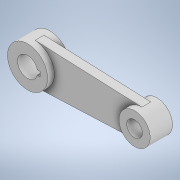
# Autodesk Inventor part: Biela da Valvula
Saved by Autodesk Inventor 2020 (Build 240168000, 168)
## iProperties
Created: 2022-04-28
Part Number: Biela da Valvula
Material: Genérico
Document SubType Name: Modeling
Designer: robofei
Density: 1 g/cm^3
Appearance: Padrão
Author: robofei
Autodesk Inventor part; units mm, degrees
ref_plane "YZ Plane" through (0, 0, 0) normal (1, 0, 0) x (0, 1, 0)
ref_plane "XZ Plane" through (0, 0, 0) normal (0, 1, 0) x (-1, 0, 0)
ref_plane "XY Plane" through (0, 0, 0) normal (0, 0, 1) x (1, 0, 0)
sketch "Esboço1" plane through (0, 0, 0) normal (0, 0, 1) x (1, 0, 0)
  circle A0 centre (0, 0) radius 21.9
  circle A1 centre (0, 0) radius 43.75
  arc A2 (-272.718, 6.3) -> (-272.718, -6.3) centre (-300, 0) ccw
  circle A3 centre (-300, 0) radius 56.25
  line L0 (-272.718, 6.3) -> (-265, 6.3)
  line L1 (-265, 6.3) -> (-265, -6.3)
  line L2 (-265, -6.3) -> (-272.718, -6.3)
  dimension "d0" = 300
  dimension "d1" = 87.5
  dimension "d2" = 43.8
  dimension "d3" = 112.5
  dimension "d4" = 56
  dimension "d6" = 12.6
  dimension "d7" = 6.3
  dimension "d8" = 35
  constraints: 6 end point, 4 centre point, 3 coincident, 2 point on circle, 1 horizontal, 1 parallel, 1 perpendicular
  measures "d0" distance of A2.centre point (0, 0)
  measures "d1" diameter of A1
  measures "d2" diameter of A0
  measures "d3" diameter of A3
  measures "d4" diameter of A2
  measures "d6" distance of L0.end L1.end
  measures "d7" distance from line of A2.centre L2
  measures "d8" horizontal distance of A2.centre L1.end
extrude "Extrusão1" add sketch "Esboço1" along normal mid plane 62.5
sketch "Esboço2" plane through (0, 0, 0) normal (0, 0, 1) x (1, 0, 0)
  arc A0 (1.8229, 43.712) -> (1.8229, -43.712) centre (0, 0) ccw
  arc A1 (-272.718, 6.3) -> (-272.718, -6.3) centre (-300, 0) ccw projected
  arc A2 (-297.6562, -56.2012) -> (-297.6562, 56.2012) centre (-300, 0) ccw
  line L0 (-297.6562, 56.2012) -> (1.8229, 43.712)
  line L1 (-297.6562, -56.2012) -> (1.8229, -43.712)
  circle A3 centre (0, 0) radius 43.75 projected
  circle A4 centre (-300, 0) radius 56.25 projected
  dimension "d11" = 87.5
  dimension "d12" = 112.5
  constraints: 4 end point, 4 point on circle, 4 tangent, 2 centre point, 2 coincident
  measures "d11" diameter of A0
  measures "d12" diameter of A2
extrude "Extrusão2" add sketch "Esboço2" along normal mid plane 25 contours A0 L1 A2 L0
